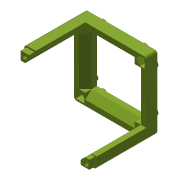
# Autodesk Inventor part: 10_Cube_base
Saved by Autodesk Inventor 2022 (Build 260153000, 153)
## iProperties
Created: 2019-07-01
Part Number: 10_Cube_base
Material: Generic
Document SubType Name: Modeling
Designer: diederichbenedict
Density: 1 g/cm^3
Appearance: IPHT_Grün
Mass: 12.3455 g
Surface Area: 84.4331 cm^2
Volume: 12.3455 cm^3
Catalog Web Link: isInjectionmolded
Vendor: openUC2
User Status: 2
Author: diederichbenedict
Autodesk Inventor part; units mm, degrees
sketch "Sketch1" plane through (0, 0, 0) normal (0, 0, 1) x (1, 0, 0)
  line L0 (-24.9, 24.9) -> (24.9, 24.9)
  line L1 (24.9, 24.9) -> (24.9, -24.9)
  line L2 (24.9, -24.9) -> (-24.9, -24.9)
  line L3 (-24.9, -24.9) -> (-24.9, 24.9)
  line L4 (-24.9, 24.9) -> (24.9, -24.9) construction
  line L5 (24.9, 24.9) -> (-24.9, -24.9) construction
  line L6 (17.02, 17.02) -> (-17.02, 17.02)
  line L7 (-17.02, 17.02) -> (-17.02, -17.02)
  line L8 (-17.02, -17.02) -> (17.02, -17.02)
  line L9 (17.02, -17.02) -> (17.02, 17.02)
  point P0 (0, 0)
  dimension "d0" = 49.8
  dimension "d1" = 49.8
  dimension "d2" = 7.88
  constraints: 20 end point, 4 parallel, 2 midpoint, 2 perpendicular, 1 horizontal, 3 other
  measures "d0" distance of L1.end L2.end
  measures "d1" distance of L0.end L1.end
  measures "d2" distance between parallel lines of L0 L6
extrude "Extrusion1" add sketch "Sketch1" along normal blind 8
sketch "Sketch2" plane through (0, 0, 8) normal (0, 0, 1) x (1, 0, 0)
  line L0 (17.02, 17.02) -> (17.02, -17.02) projected
  line L1 (17.02, -17.02) -> (-17.02, -17.02) projected
  line L2 (-17.02, -17.02) -> (-17.02, 17.02) projected
  line L3 (-17.02, 17.02) -> (17.02, 17.02) projected
  line L4 (24.9, 24.9) -> (-24.9, 24.9) projected
  line L5 (-24.9, 24.9) -> (-24.9, -24.9) projected
  line L6 (-24.9, -24.9) -> (24.9, -24.9) projected
  line L7 (24.9, -24.9) -> (24.9, 24.9) projected
  line L8 (17.02, -17.02) -> (24.9, -17.02)
  line L9 (24.9, -17.02) -> (24.9, -24.9)
  line L10 (24.9, -24.9) -> (17.02, -24.9)
  line L11 (17.02, -24.9) -> (17.02, -17.02)
  line L12 (17.02, 17.02) -> (-17.02, 17.02) projected
  line L13 (24.9, 24.9) -> (17.02, 24.9)
  line L14 (17.02, 24.9) -> (17.02, 17.02)
  line L15 (17.02, 17.02) -> (24.9, 17.02)
  line L16 (24.9, 17.02) -> (24.9, 24.9)
  line L17 (-24.9, -24.9) -> (-17.02, -24.9)
  line L18 (-17.02, -24.9) -> (-17.02, -17.02)
  line L19 (-17.02, -17.02) -> (-24.9, -17.02)
  line L20 (-24.9, -17.02) -> (-24.9, -24.9)
  line L21 (-24.9, 24.9) -> (-17.02, 24.9)
  line L22 (-17.02, 24.9) -> (-17.02, 17.02)
  line L23 (-17.02, 17.02) -> (-24.9, 17.02)
  line L24 (-24.9, 17.02) -> (-24.9, 24.9)
  point P0 (0, 0)
  constraints: 32 end point, 8 parallel, 4 horizontal, 4 perpendicular
extrude "Extrusion2" add sketch "Sketch2" along normal blind 34.1 contours L8 L7 L6 L11 | L23 L5 L4 L22
sketch "Sketch3" plane through (0, 0, 0) normal (0, 0, -1) x (-1, 0, 0)
  line L0 (24.9, -24.9) -> (24.9, 24.9) construction
  line L1 (24.9, 24.9) -> (-24.9, 24.9) construction
  line L2 (-24.9, -24.9) -> (24.9, -24.9) construction
  line L3 (-24.9, 24.9) -> (-24.9, -24.9) construction
  line L4 (-17.02, -17.02) -> (-17.02, 17.02) projected
  line L5 (-17.02, 17.02) -> (17.02, 17.02) projected
  line L6 (17.02, 17.02) -> (17.02, -17.02) projected
  line L7 (17.02, -17.02) -> (-17.02, -17.02) projected
  line L8 (24.9, 24.9) -> (-24.9, 24.9) projected
  line L9 (-24.9, 24.9) -> (-24.9, -24.9) projected
  line L10 (-24.9, -24.9) -> (24.9, -24.9) projected
  line L11 (24.9, -24.9) -> (24.9, 24.9) projected
  point P0 (21.25, 21.25)
  point P1 (21.25, -21.25)
  point P2 (-21.25, -21.25)
  point P3 (-21.25, 21.25)
  dimension "d_1" = 3.65
  dimension "d96" = 3.65
  dimension "d97" = 3.65
  dimension "d98" = 3.65
  dimension "d99" = 3.65
  dimension "d100" = 3.65
  dimension "d101" = 3.65
  dimension "d102" = 3.65
  measures "d_1" distance from line of L1 point (21.25, 21.25)
  measures "d96" distance from line of point (21.25, 21.25) L0
  measures "d97" distance from line of point (21.25, -21.25) L0
  measures "d98" distance from line of point (21.25, -21.25) L2
  measures "d99" distance from line of point (-21.25, -21.25) L2
  measures "d100" distance from line of point (-21.25, -21.25) L3
  measures "d101" distance from line of point (-21.25, 21.25) L3
  measures "d102" distance from line of point (-21.25, 21.25) L1
hole "Hole1" at (-21.25, 21.25, 0) at (21.25, -21.25, 0) direction (0, 0, 1) diameter 3.1 end through all counterbore diameter 5.5 counterbore depth 4.6
sketch "Sketch6" plane through (0, 0, 42.1) normal (0, 0, 1) x (1, 0, 0)
  line L0 (-24.9, 24.9) -> (-24.9, 17.02)
  line L1 (-24.9, 17.02) -> (-17.02, 17.02)
  line L2 (-17.02, 17.02) -> (-17.02, 24.9)
  line L3 (-17.02, 24.9) -> (-24.9, 24.9)
  line L4 (24.9, -24.9) -> (24.9, -17.02)
  line L5 (24.9, -17.02) -> (17.02, -17.02)
  line L6 (17.02, -17.02) -> (17.02, -24.9)
  line L7 (17.02, -24.9) -> (24.9, -24.9)
  line L8 (0, 38.183766) -> (54, 38.183766) construction
  line L9 (-17.02, 24.9) -> (-17.02, 17.02)
  line L10 (-17.02, 17.02) -> (-17.02, 21.268615)
  line L11 (-17.02, 21.268615) -> (-21.271053, 17.02)
  line L12 (-17.02, 21.268615) -> (-11.009827, 21.268615) construction
  line L13 (-21.271053, 17.02) -> (-17.02, 17.02)
  line L14 (-17.02, 17.02) -> (-21.271053, 17.02)
  line L15 (17.02, -17.02) -> (17.02, -24.9)
  line L16 (17.02, -17.02) -> (21.271053, -17.02)
  line L17 (24.9, -17.02) -> (17.02, -17.02)
  line L18 (21.271053, -17.02) -> (17.02, -21.268615)
  line L19 (17.02, -17.02) -> (17.02, -21.268615)
  line L20 (17.02, -17.02) -> (24.9, -17.02)
  line L21 (24.9, -17.02) -> (24.9, 24.9)
  line L22 (24.9, 24.9) -> (-17.02, 24.9)
  line L23 (-17.02, 24.9) -> (-17.02, 17.02)
  line L24 (-17.02, 17.02) -> (17.02, 17.02) construction
  line L25 (17.02, 17.02) -> (17.02, -17.02) construction
  line L26 (17.02, -24.9) -> (17.02, -17.02)
  line L27 (17.02, -17.02) -> (-17.02, -17.02)
  line L28 (-17.02, -17.02) -> (-17.02, 17.02)
  line L29 (-17.02, 17.02) -> (-24.9, 17.02)
  line L30 (-24.9, 17.02) -> (-24.9, -24.9)
  line L31 (-24.9, -24.9) -> (17.02, -24.9)
  circle A0 centre (0, 0) radius 17.02
  line L32 (-0.010984, -38.289831) -> (38.289831, -0.010984) construction
  line L33 (38.289831, -0.010984) -> (0.010984, 38.289831) construction
  line L34 (0.010984, 38.289831) -> (-38.289831, 0.010984) construction
  line L35 (-38.289831, 0.010984) -> (-0.010984, -38.289831) construction
  line L36 (-0.010984, -38.289831) -> (0.010984, 38.289831) construction
  line L37 (38.289831, -0.010984) -> (-38.289831, 0.010984) construction
  point P0 (0, 0)
  point P1 (0, 0)
  dimension "d192" = 54.15
  dimension "d193" = 54.15
  dimension "d194" = 0
  dimension "d195" = 0
  constraints: 30 end point, 4 point on line, 3 collinear, 3 midpoint, 3 parallel, 3 tangent, 2 horizontal, 1 centre point, 1 coincident, 1 equal length, 1 perpendicular
  measures "d192" distance of L32.start L32.end
  measures "d193" distance of L33.end L32.end
  measures "d194" distance between parallel lines of L34 L11
  measures "d195" distance between parallel lines of L32 L18
extrude "Extrusion3" cut sketch "Sketch6" against normal up to surface (34.1 mm away) contours L11 L2 L1 | L6 L5 L18
sketch "Sketch7" plane through (-24.9, 17.02, 8) normal (0, -1, 0) x (1, 0, 0)
  line L0 (41.92, 0) -> (49.92, 0) construction
  line L1 (41.92, -8) -> (41.92, 0) construction
  line L2 (7.88, -8.035061) -> (7.88, 0) construction
  line L3 (-0.12, 0) -> (7.88, 0) construction
  line L4 (46.169832, 0) -> (41.92, 0)
  line L5 (46.169832, 0) -> (41.92, -4.249832)
  line L6 (41.92, 0) -> (41.92, -4.249832)
  line L7 (46.169832, 0) -> (41.92, 0)
  line L8 (41.92, 0) -> (46.169832, 0)
  line L9 (7.88, 0) -> (3.630168, 0)
  line L10 (3.630168, 0) -> (7.88, -4.249832)
  line L11 (7.88, -4.249832) -> (7.88, 0)
  line L12 (41.92, 0) -> (7.88, 0) construction
  line L13 (7.88, 0) -> (7.88, 34.1) construction
  line L14 (41.92, 34.1) -> (41.92, 0) construction
  circle A0 centre (24.9, 17.02) radius 17.02 construction
  line L15 (24.9, 55.309832) -> (63.189832, 17.02) construction
  line L16 (63.189832, 17.02) -> (24.9, -21.269832) construction
  line L17 (24.9, -21.269832) -> (-13.389832, 17.02) construction
  line L18 (-13.389832, 17.02) -> (24.9, 55.309832) construction
  line L19 (24.9, 55.309832) -> (24.9, -21.269832) construction
  line L20 (63.189832, 17.02) -> (-13.389832, 17.02) construction
  line L21 (24.9, 55.309832) -> (79.05, 55.309832) construction
  point P0 (44.385994, 0)
  point P1 (43.597772, 0)
  dimension "d187" = 54.15
  dimension "d188" = 45
  dimension "d189" = 54.15
  dimension "d190" = 135
  dimension "d191" = 135
  constraints: 36 end point, 6 point on line, 3 collinear, 3 tangent, 2 midpoint, 2 parallel, 1 centre point, 1 equal length, 1 horizontal, 1 perpendicular, 1 vertical
  measures "d187" distance of L15.start L15.end
  measures "d188" angle of L15 L21
  measures "d189" distance of L15.end L16.end
  measures "d190" angle of L5 L4
  measures "d191" angle of L17 L11
extrude "Extrusion4" cut sketch "Sketch7" along normal up to surface (34.04 mm away)
sketch "Sketch8" plane through (17.02, -24.9, 8) normal (-1, 0, 0) x (0, 0, 1)
  line L0 (-4.18, 41.92) -> (0, 41.92) construction
  line L1 (-4.18, 7.88) -> (0, 7.88) construction
  line L2 (0, 7.88) -> (0, 3.7) construction
  line L3 (-4.18, 7.88) -> (0, 3.7)
  line L4 (0, 3.7) -> (0, 7.88)
  line L5 (0, 7.88) -> (-4.18, 7.88)
  line L6 (-4.18, 41.92) -> (0, 46.1)
  line L7 (-4.18, 41.92) -> (1.731413, 41.92) construction
  line L8 (0, 7.88) -> (0, 41.92)
  line L9 (0, 46.1) -> (0, 41.92)
  line L10 (0, 41.92) -> (-4.18, 41.92)
  line L11 (-5.97417, 2.086412) -> (-5.97417, 47.213342)
  line L12 (-8, 49.8) -> (-8, 0) construction
  line L13 (-8, 49.8) -> (0, 49.8) construction
  line L14 (0, 7.88) -> (0, 49.8) construction
  line L15 (0, 7.88) -> (34.1, 7.88) construction
  line L16 (34.1, 0) -> (34.1, 7.88) construction
  line L17 (-8, 0) -> (34.1, 0) construction
  line L18 (0, 0) -> (0, 3.631385) construction
  line L19 (0, 7.88) -> (0, 3.631385) construction
  line L20 (0, 49.8) -> (0, 46.168615) construction
  line L21 (0, 41.92) -> (0, 7.88)
  line L22 (0, 7.88) -> (0, 49.8)
  line L23 (0, 49.8) -> (0, 46.168615)
  line L24 (0, 41.92) -> (0, 46.168615)
  line L25 (0, 7.88) -> (0, 41.92)
  line L26 (0, 41.92) -> (0, 0)
  point P0 (-2.460709, 7.998236)
  point P1 (-0.062345, 5.450246)
  dimension "d112" = 45
  dimension "d181" = 4.18
  dimension "d182" = 4.18
  dimension "d183" = 4.18
  constraints: 20 end point, 3 horizontal, 2 vertical, 1 collinear, 1 equal length, 1 perpendicular, 6 other
  measures "d112" angle of L7 L6
  measures "d181" distance of L3.start L4.end
  measures "d182" distance of L3.end L4.end
  measures "d183" distance of L0.end L0.start
ref_plane "Work Plane1" through (-20.32, -18.034, 19.81812) normal (-1, 0, 0) x (0, 0, 1)
extrude "Extrusion5" cut sketch "Sketch8" along normal up to surface (34.04 mm away)
sketch "Sketch17" plane through (0, 0, 42.1) normal (0, 0, 1) x (1, 0, 0)
  circle A0 centre (-21.25, 21.25) radius 2.75 construction
  line L0 (-21.271053, 17.02) -> (-17.02, 21.268615) construction
  line L1 (-17.02, 21.268615) -> (-17.02, 24.9) construction
  line L2 (-17.02, 24.9) -> (-24.9, 24.9) construction
  line L3 (-24.9, 24.9) -> (-24.9, 17.02) construction
  line L4 (-24.9, 17.02) -> (-21.271053, 17.02) construction
  line L5 (21.271053, -17.02) -> (17.02, -21.268615) construction
  line L6 (17.02, -21.268615) -> (17.02, -24.9) construction
  line L7 (17.02, -24.9) -> (24.9, -24.9) construction
  line L8 (24.9, -24.9) -> (24.9, -17.02) construction
  line L9 (24.9, -17.02) -> (21.271053, -17.02) construction
  line L10 (-20.590663, 17.7) -> (-23.8, 17.7)
  line L11 (-23.8, 17.7) -> (-23.8, 23.8)
  line L12 (-23.8, 23.8) -> (-17.7, 23.8)
  line L13 (-17.7, 23.8) -> (-17.7, 20.589005)
  line L14 (-21.271053, 17.02) -> (-17.02, 21.268615)
  line L15 (-20.590663, 17.7) -> (-17.7, 20.589005)
  line L16 (-20.956009, -20.943989) -> (20.956009, 20.943989) construction
  circle A1 centre (21.237805, -21.262188) radius 2.75 construction
  circle A2 centre (21.2, -21.2) radius 1.4
  line L17 (17.02, -21.268615) -> (21.271053, -17.02) construction
  line L18 (21.271053, -17.02) -> (24.9, -17.02) construction
  line L19 (24.9, -17.02) -> (24.9, -24.9) construction
  line L20 (24.9, -24.9) -> (17.02, -24.9) construction
  line L21 (17.02, -24.9) -> (17.02, -21.268615) construction
  line L22 (17.688184, -20.600815) -> (17.686342, -23.810151)
  line L23 (17.686342, -23.810151) -> (23.786341, -23.813651)
  line L24 (23.786341, -23.813651) -> (23.789841, -17.713652)
  line L25 (23.789841, -17.713652) -> (20.578847, -17.711809)
  line L26 (17.02, -21.268615) -> (21.271053, -17.02)
  line L27 (17.688184, -20.600815) -> (20.578847, -17.711809)
  circle A3 centre (-21.25, 21.25) radius 1.55
  circle A4 centre (21.25, -21.25) radius 1.55
  point P0 (0, 0)
  dimension "d171" = 6.1
  dimension "d172" = 6.1
  dimension "d173" = 1.1
  dimension "d174" = 1.1
  constraints: 34 end point, 6 symmetric about line, 4 point on line, 3 perpendicular, 2 centre point, 1 collinear, 1 horizontal, 1 other
  measures "d171" distance between parallel lines of L12 L10
  measures "d172" distance between parallel lines of L13 L11
  measures "d173" distance between parallel lines of L3 L11
  measures "d174" distance between parallel lines of L2 L12
extrude "Extrusion7" add sketch "Sketch17" along normal blind 3.7 contours L10 L11 L12 L13 L14 | L26 L25 L24 L23 L22
sketch "Sketch18" plane through (0, 0, 8) normal (0, 0, 1) x (1, 0, 0)
  line L0 (20.672698, 17.65) -> (23.75, 17.65)
  line L1 (23.75, 17.65) -> (23.75, 23.75)
  line L2 (23.75, 23.75) -> (17.65, 23.75)
  line L3 (17.65, 23.75) -> (17.65, 20.970419)
  line L4 (17.65, 20.970419) -> (20.672698, 17.65)
  circle A0 centre (21.2, 21.2) radius 1.55
  line L5 (-17.65, -20.672698) -> (-17.65, -23.75)
  line L6 (-17.65, -23.75) -> (-23.75, -23.75)
  line L7 (-23.75, -23.75) -> (-23.75, -17.65)
  line L8 (-23.75, -17.65) -> (-20.970419, -17.65)
  line L9 (-20.970419, -17.65) -> (-17.65, -20.672698)
  circle A1 centre (-21.2, -21.2) radius 1.55
  dimension "d164" = 3.1
  dimension "d169" = 6.1
  dimension "d170" = 6.1
  constraints: 20 end point, 2 centre point
  measures "d164" diameter of A0
  measures "d169" distance between parallel lines of L3 L1
  measures "d170" distance between parallel lines of L2 L0
extrude "Extrusion8" cut sketch "Sketch18" against normal blind 4.2 contours L4 L3 L2 L1 L0 | A0 | L5 L6 L7 L8 L9 | A1
fillet "Fillet2" radius 2 4 edges at (24.9, -24.9, 21.05) (24.9, 24.9, 4) (-24.9, 24.9, 21.05) (-24.9, -24.9, 4)
fillet "Fillet2" radius 0.5 24 edges at (23.7898, -17.7137, 43.95) (23.7863, -23.8137, 43.95) (20.5788, -17.7118, 43.95) (-17.7, 23.8, 43.95) (-17.7, 20.589, 43.95) (-23.8, 23.8, 43.95) (-23.8, 17.7, 43.95) (-20.5907, 17.7, 43.95) (17.6882, -20.6008, 43.95) (17.6863, -23.8102, 43.95) (23.75, 23.75, 5.9) (20.6727, 17.65, 5.9) (17.65, 20.9704, 5.9) (17.65, 23.75, 5.9) (23.75, 17.65, 5.9) (0, 24.9, 0) (24.9, 0, 0) (-24.9, 0, 0) (0, -24.9, 0) (-20.9704, -17.65, 5.9) (-23.75, -17.65, 5.9) (-17.65, -20.6727, 5.9) (-17.65, -23.75, 5.9) (-23.75, -23.75, 5.9)
sketch "Sketch20" plane through (0, 0, 0) normal (0, 0, -1) x (-1, 0, 0)
  line L0 (-17.02, -17.02) -> (-17.02, 17.02) construction
  line L1 (-17.02, 17.02) -> (17.02, 17.02) construction
  line L2 (17.02, 17.02) -> (17.02, -17.02) construction
  line L3 (17.02, -17.02) -> (-17.02, -17.02) construction
  circle A0 centre (21.25, 21.25) radius 2.75 construction
  circle A1 centre (-21.25, -21.25) radius 2.75 construction
  arc A2 (-24.4, -22.9) -> (-22.9, -24.4) centre (-22.9, -22.9) ccw construction
  line L4 (22.9, -24.4) -> (-22.9, -24.4) construction
  arc A3 (22.9, -24.4) -> (24.4, -22.9) centre (22.9, -22.9) ccw construction
  line L5 (24.4, 22.9) -> (24.4, -22.9) construction
  arc A4 (24.4, 22.9) -> (22.9, 24.4) centre (22.9, 22.9) ccw construction
  line L6 (-22.9, 24.4) -> (22.9, 24.4) construction
  arc A5 (-22.9, 24.4) -> (-24.4, 22.9) centre (-22.9, 22.9) ccw construction
  line L7 (-24.4, -22.9) -> (-24.4, 22.9) construction
  circle A6 centre (-14.3, 20.71) radius 2.475
  circle A7 centre (-14.3, 20.71) radius 1.025 construction
  line L8 (8.8, 20.71) -> (-17.124859, 20.71) construction
  line L9 (0, -34.86) -> (0, 34.86) construction
  circle A8 centre (14.3, 20.71) radius 2.475
  circle A9 centre (14.3, 20.71) radius 1.025 construction
  circle A10 centre (-20.71, -14.3) radius 1.025 construction
  circle A11 centre (-20.71, -14.3) radius 2.475
  circle A12 centre (-20.71, 14.3) radius 1.025 construction
  circle A13 centre (-20.71, 14.3) radius 2.475
  circle A14 centre (14.3, -20.71) radius 1.025 construction
  circle A15 centre (14.3, -20.71) radius 2.475
  circle A16 centre (-14.3, -20.71) radius 1.025 construction
  circle A17 centre (-14.3, -20.71) radius 2.475
  circle A18 centre (20.71, 14.3) radius 1.025 construction
  circle A19 centre (20.71, 14.3) radius 2.475
  circle A20 centre (20.71, -14.3) radius 1.025 construction
  circle A21 centre (20.71, -14.3) radius 2.475
  point P0 (0, 0)
  point P1 (-8.8, 20.71)
  point P2 (17.124859, 20.71)
  point P3 (-20.71, -17.124859)
  point P4 (-20.71, 17.124859)
  point P5 (17.124859, -20.71)
  point P6 (-17.124859, -20.71)
  point P7 (20.71, 17.124859)
  point P8 (20.71, -17.124859)
  dimension "d144" = 4.95
  dimension "d145" = 2.05
  dimension "d146" = 5.5
  dimension "d149" = 360
  constraints: 16 centre point, 8 coincident, 3 symmetric about line, 2 end point, 2 point on line, 1 horizontal, 43 other
  measures "d144" diameter of A6
  measures "d145" diameter of A7
  measures "d146" distance of point (-8.8, 20.71) A6.centre
extrude "Extrusion10" add sketch "Sketch20" along normal blind 2.2 draft -2
ref_plane "Work Plane2" through (0, -17.02, 42.1) normal (1, 0, 0) x (0, 0, -1)
ref_plane "Work Plane3" through (-17.02, 0, 42.1) normal (0, 1, 0) x (1, 0, 0)
ref_plane "Work Plane4" through (-24.9, 24.9, 8) normal (-0.7071068, -0.7071068, 0) x (0, 0, 1)
equation "\"d96\" = d_1"
equation "\"d97\" = d_1"
equation "\"d98\" = d_1"
equation "\"d99\" = d_1"
equation "\"d100\" = d_1"
equation "\"d101\" = d_1"
equation "\"d102\" = d_1"
body "Solid1"
